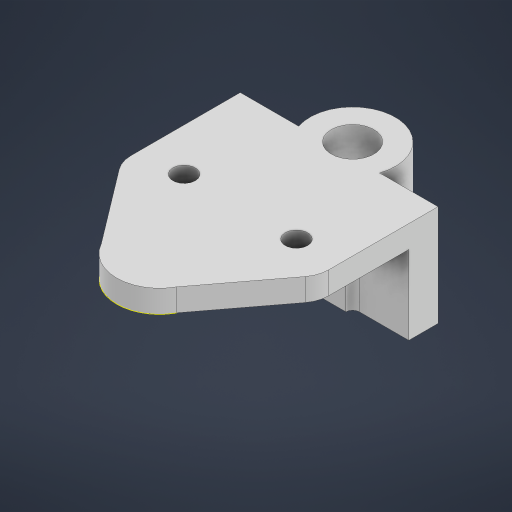
# Autodesk Inventor part: Część10
Saved by Autodesk Inventor 2023 (Build 270158000, 158)
## iProperties
Created: 2023-05-07
Part Number: Część10
Material: Ogólny
Document SubType Name: Modeling
Designer: Adam
Density: 1 g/cm^3
Appearance: Domyślna
Author: Adam
Autodesk Inventor part; units mm, degrees
ref_plane "YZ Plane" through (0, 0, 0) normal (1, 0, 0) x (0, 1, 0)
ref_plane "XZ Plane" through (0, 0, 0) normal (0, 1, 0) x (-1, 0, 0)
ref_plane "XY Plane" through (0, 0, 0) normal (0, 0, 1) x (1, 0, 0)
sketch "Szkic1" plane through (0, 0, 0) normal (0, 1, 0) x (-1, 0, 0)
  circle A0 centre (0, -95.1906) radius 19
  line L0 (-44, -89.1906) -> (44, -89.1906)
  line L1 (44, -89.1906) -> (44, -76.1906)
  line L2 (44, -76.1906) -> (-44, -76.1906)
  line L3 (-44, -76.1906) -> (-44, -89.1906)
  line L4 (-19, -76.1906) -> (19, -76.1906)
  line L5 (19, -76.1906) -> (19, -73.1906)
  line L6 (19, -73.1906) -> (-19, -73.1906)
  line L7 (-19, -73.1906) -> (-19, -76.1906)
  point P0 (0, 0)
  point P1 (0, -76.1906)
  point P2 (0, -76.1906)
  point P3 (0, -74.6906)
  point P4 (-18.0278, -89.1906)
  point P5 (18.0278, -89.1906)
  dimension "d0" = 38
  dimension "d1" = 88
  dimension "d2" = 13
  dimension "d3" = 38
  dimension "d4" = 3
  constraints: 16 end point, 4 parallel, 2 horizontal, 2 perpendicular, 2 point on circle, 1 centre point, 1 collinear, 1 midpoint
  measures "d0" diameter of A0
  measures "d1" distance of L2.end L1.end
  measures "d2" distance of L1.end L0.end
  measures "d3" distance of L6.end L5.end
  measures "d4" distance of L5.end L4.end
extrude "Wyciągnięcie proste1" add sketch "Szkic1" along normal blind 45
sketch "Szkic2" plane through (0, 45, 0) normal (0, 1, 0) x (1, 0, 0)
  line L0 (-44, 76.1906) -> (44, 76.1906)
  line L1 (44, 76.1906) -> (44, 40.5529)
  line L2 (-44, 40.5529) -> (-44, 76.1906)
  circle A0 centre (0, 9.1906) radius 19
  line L3 (41.3686, 32.7112) -> (16.6293, 0)
  line L4 (-41.3686, 32.7112) -> (-16.6293, 0)
  arc A1 (-44, 40.5529) -> (-41.3686, 32.7112) centre (-31, 40.5529) ccw
  arc A2 (41.3686, 32.7112) -> (44, 40.5529) centre (31, 40.5529) ccw
  point P0 (0, 0)
  point P1 (44, 36.1906)
  point P2 (-44, 36.1906)
  point P3 (-25, 45.1906)
  point P4 (25, 45.1906)
  dimension "d7" = 88
  dimension "d8" = 40
  dimension "d9" = 31
  dimension "d10" = 19
  dimension "d11" = 38
  dimension "d13" = 36
  dimension "d14" = 13
  dimension "d15" = 13
  constraints: 10 end point, 6 point on circle, 4 point on line, 4 tangent, 3 centre point, 1 horizontal, 1 parallel, 1 perpendicular
  measures "d7" distance of point (44, 36.191) point (-44, 36.191)
  measures "d8" distance of L0.end point (44, 36.191)
  measures "d9" distance from line of L0 point (-25, 45.191)
  measures "d10" distance from line of L2 point (-25, 45.191)
  measures "d11" diameter of A0
  measures "d13" vertical distance of A0.centre point (25, 45.191)
  measures "d14" radius of A1
  measures "d15" radius of A2
extrude "Wyciągnięcie proste2" add sketch "Szkic2" against normal blind 10
fillet "Zaokrąglenie1" radius 3 1 edges at (19, 17.5, -76.1906)
fillet "Zaokrąglenie2" radius 3 1 edges at (-19, 17.5, -76.1906)
sketch "Szkic3" plane through (0, 35, 0) normal (0, -1, 0) x (1, 0, 0)
  arc A0 (16.6293, 0) -> (-16.6293, 0) centre (0, -9.1906) ccw projected
  point P0 (0, 0)
sketch "Szkic4" plane through (0, 0, 0) normal (0, -1, 0) x (1, 0, 0)
  arc A0 (-18.0278, -89.1906) -> (18.0278, -89.1906) centre (0, -95.1906) ccw projected
  point P0 (0, 0)
  constraints: 1 coincident
hole "Otwór1" at (0, 0, -95.1906) direction (0, 1, 0) diameter 19 end through all
sketch "Szkic5" plane through (0, 35, 0) normal (0, -1, 0) x (1, 0, 0)
  line L0 (22, -76.1906) -> (44, -76.1906) projected
  line L1 (44, -76.1906) -> (44, -40.5529) projected
  point P0 (0, 0)
  point P1 (25, -45.1906)
  point P2 (-25, -45.1906)
  dimension "d27" = 31
  dimension "d28" = 19
  measures "d27" distance from line of L0 point (25, -45.191)
  measures "d28" distance from line of point (25, -45.191) L1
hole "Otwór2" at (25, 35, -45.1906) at (-25, 35, -45.1906) direction (0, 1, 0) diameter 10 end through all
sketch "Szkic6" plane through (0, 0, 0) normal (1, 0, 0) x (0, 1, 0)
  line L0 (0, -73.1906) -> (0, -69.1906)
  line L1 (0, -69.1906) -> (35, -9.1906)
  line L2 (35, -32.7112) -> (35, 0) projected
  point P0 (0, 0)
  point P1 (35, -76.1906)
  dimension "d36" = 4
  dimension "d37" = 67
  constraints: 4 end point, 1 point on line, 1 vertical
  measures "d36" distance of L0.start L0.end
  measures "d37" distance of L1.end point (35, -76.191)
extrude "Żebro1" add sketch "Szkic6" along normal mid plane 10 rib yes fills toward (0.05, -71.1906) open curves L0 L1
